Autodesk Fusion 360 part; units mm, degrees
note: some values were not read from the file. Set by a fixed rule: which sketch regions a step uses.
(part 4 of 4)
  line L683 (3.4369, -40.79) -> (3.9769, -40.4465)
  line L684 (3.9769, -40.4465) -> (3.9994, -40.4318)
  line L685 (3.9994, -40.4318) -> (4.2354, -40.3019)
  line L686 (4.2354, -40.3019) -> (4.2599, -40.2908)
  line L687 (4.2599, -40.2908) -> (4.2279, -40.2967)
  line L688 (4.2279, -40.2967) -> (3.9619, -40.3254)
  line L689 (3.9619, -40.3254) -> (3.4369, -40.3254)
  line L690 (3.4369, -40.3254) -> (3.4369, -39.957)
  line L691 (3.4369, -39.957) -> (4.9125, -39.9578)
  line L692 (4.9125, -39.9578) -> (4.9125, -40.3262)
  line L693 (4.9125, -40.3262) -> (4.2619, -40.7299)
  line L694 (4.2619, -40.7299) -> (4.2373, -40.7447)
  line L695 (4.2373, -40.7447) -> (3.9836, -40.8754)
  line L696 (3.777, -41.5549) -> (3.777, -42.2201)
  line L697 (3.777, -42.2201) -> (3.9912, -42.2201)
  line L698 (3.9912, -42.2201) -> (3.9912, -41.6824)
  line L699 (3.9912, -41.6824) -> (4.3186, -41.6824)
  line L700 (4.3186, -41.6824) -> (4.3186, -42.2201)
  line L701 (4.3186, -42.2201) -> (4.5619, -42.2201)
  line L702 (4.5619, -42.2201) -> (4.5619, -41.5549)
  line L703 (4.5619, -41.5549) -> (4.9141, -41.5549)
  line L704 (4.9141, -41.5549) -> (4.9141, -42.665)
  line L705 (4.9141, -42.665) -> (3.4369, -42.665)
  line L706 (3.4369, -42.665) -> (3.4369, -41.5549)
  line L707 (3.4369, -41.5549) -> (3.777, -41.5549)
  line L708 (4.9125, -44.0314) -> (3.4369, -44.0314)
  line L709 (3.4369, -44.0314) -> (3.4369, -42.965)
  line L710 (3.4369, -42.965) -> (3.7879, -42.965)
  line L711 (3.7879, -42.965) -> (3.7879, -43.5908)
  line L712 (3.7879, -43.5908) -> (4.0279, -43.5908)
  line L713 (4.0279, -43.5908) -> (4.0279, -43.1102)
  line L714 (4.0279, -43.1102) -> (4.3606, -43.1102)
  line L715 (4.3606, -43.1102) -> (4.3606, -43.5908)
  line L716 (4.3606, -43.5908) -> (4.9125, -43.5908)
  line L717 (4.9125, -43.5908) -> (4.9125, -44.0314)
  line L718 (4.2994, -45.1875) -> (4.2994, -44.949)
  line L719 (4.2994, -44.949) -> (3.8715, -45.0684)
  line L720 (3.8715, -45.0684) -> (4.2994, -45.1875)
  line L721 (4.9125, -44.7863) -> (4.6219, -44.8695)
  line L722 (4.6219, -44.8695) -> (4.6219, -45.2648)
  line L723 (4.6219, -45.2648) -> (4.9125, -45.3533)
  line L724 (4.9125, -45.3533) -> (4.9125, -45.7209)
  line L725 (4.9125, -45.7209) -> (3.4369, -45.2656)
  line L726 (3.4369, -45.2656) -> (3.4369, -44.7867)
  line L727 (3.4369, -44.7867) -> (4.9113, -44.3244)
  line L728 (4.9113, -44.3244) -> (4.9125, -44.7863)
  line L729 (3.9791, -46.4652) -> (3.4369, -46.4652)
  line L730 (3.4369, -46.4652) -> (3.4369, -46.0125)
  line L731 (3.4369, -46.0125) -> (4.9113, -46.0125)
  line L732 (4.9113, -46.0125) -> (4.9113, -46.4652)
  line L733 (4.9113, -46.4652) -> (4.3393, -46.4652)
  line L734 (4.3393, -46.4652) -> (4.3393, -46.8109)
  line L735 (4.3393, -46.8109) -> (4.9125, -46.8109)
  line L736 (4.9125, -46.8109) -> (4.9125, -47.2637)
  line L737 (4.9125, -47.2637) -> (3.4369, -47.2637)
  line L738 (3.4369, -47.2637) -> (3.4369, -46.8109)
  line L739 (3.4369, -46.8109) -> (3.9791, -46.8109)
  line L740 (3.9791, -46.8109) -> (3.9791, -46.4652)
  line L741 (4.0338, -48.2893) -> (4.0039, -48.1742)
  line L742 (4.0039, -48.1742) -> (3.9975, -48.1639)
  line L743 (3.9975, -48.1639) -> (3.9916, -48.1553)
  line L744 (3.9916, -48.1553) -> (3.952, -48.1244)
  line L745 (3.952, -48.1244) -> (3.9033, -48.1117)
  line L746 (3.9033, -48.1117) -> (3.893, -48.1121)
  line L747 (3.893, -48.1121) -> (3.8662, -48.1121)
  line L748 (3.8662, -48.1121) -> (3.7865, -48.1557)
  line L749 (3.7865, -48.1557) -> (3.7512, -48.2533)
  line L750 (3.7512, -48.2533) -> (3.7512, -48.4943)
  line L751 (3.7512, -48.4943) -> (4.0332, -48.4943)
  line L752 (4.0332, -48.4943) -> (4.0332, -48.3012)
  line L753 (4.0332, -48.3012) -> (4.0338, -48.2893)
  line L754 (3.4369, -48.1211) -> (3.4666, -47.9514)
  line L755 (3.4666, -47.9514) -> (3.5363, -47.8055)
  line L756 (3.5363, -47.8055) -> (3.5563, -47.7818)
  line L757 (3.5563, -47.7818) -> (3.5755, -47.7586)
  line L758 (3.5755, -47.7586) -> (3.6973, -47.6748)
  line L759 (3.6973, -47.6748) -> (3.8408, -47.6398)
  line L760 (3.8408, -47.6398) -> (3.8711, -47.6408)
  line L761 (3.8711, -47.6408) -> (3.8906, -47.6404)
  line L762 (3.8906, -47.6404) -> (4.0787, -47.6838)
  line L763 (4.0787, -47.6838) -> (4.0961, -47.6926)
  line L764 (4.0961, -47.6926) -> (4.1123, -47.7014)
  line L765 (4.1123, -47.7014) -> (4.1879, -47.7709)
  line L766 (4.1879, -47.7709) -> (4.2559, -47.876)
  line L767 (4.2559, -47.876) -> (4.2684, -47.9021)
  line L768 (4.2684, -47.9021) -> (4.9125, -47.6344)
  line L769 (4.9125, -47.6344) -> (4.9125, -48.1361)
  line L770 (4.9125, -48.1361) -> (4.35, -48.3518)
  line L771 (4.35, -48.3518) -> (4.35, -48.4943)
  line L772 (4.35, -48.4943) -> (4.9125, -48.4943)
  line L773 (4.9125, -48.4943) -> (4.9125, -48.9469)
  line L774 (4.9125, -48.9469) -> (3.4369, -48.9469)
  line L775 (3.4369, -48.9469) -> (3.4369, -48.1211)
  line L776 (3.9912, -49.4111) -> (4.3186, -49.4111)
  line L777 (4.3186, -49.4111) -> (4.3186, -49.949)
  line L778 (4.3186, -49.949) -> (4.5619, -49.949)
  line L779 (4.5619, -49.949) -> (4.5619, -49.2838)
  line L780 (4.5619, -49.2838) -> (4.9141, -49.2838)
  line L781 (4.9141, -49.2838) -> (4.9141, -50.393)
  line L782 (4.9141, -50.393) -> (3.4369, -50.393)
  line L783 (3.4369, -50.393) -> (3.4369, -49.2838)
  line L784 (3.4369, -49.2838) -> (3.777, -49.2838)
  line L785 (3.777, -49.2838) -> (3.777, -49.949)
  line L786 (3.777, -49.949) -> (3.9912, -49.949)
  line L787 (3.9912, -49.949) -> (3.9912, -49.4111)
  line L788 (4.9125, -51.5742) -> (4.9125, -52.0025)
  line L789 (4.9125, -52.0025) -> (3.4369, -52.0025)
  line L790 (3.4369, -52.0025) -> (3.4369, -51.5758)
  line L791 (3.4369, -51.5758) -> (4.0467, -51.5758)
  line L792 (4.0467, -51.5758) -> (3.4369, -51.1678)
  line L793 (3.4369, -51.1678) -> (3.4369, -50.7607)
  line L794 (3.4369, -50.7607) -> (3.9766, -51.1332)
  line L795 (3.9766, -51.1332) -> (4.9125, -50.6713)
  line L796 (4.9125, -50.6713) -> (4.9125, -51.1666)
  line L797 (4.9125, -51.1666) -> (4.3553, -51.4213)
  line L798 (4.3553, -51.4213) -> (4.5725, -51.5742)
  line L799 (4.5725, -51.5742) -> (4.9125, -51.5742)
  line L800 (4.2994, -53.1574) -> (4.2994, -52.9185)
  line L801 (4.2994, -52.9185) -> (3.8715, -53.0379)
  line L802 (3.8715, -53.0379) -> (4.2994, -53.1574)
  line L803 (4.6219, -52.8391) -> (4.6219, -53.2344)
  line L804 (4.6219, -53.2344) -> (4.9125, -53.3228)
  line L805 (4.9125, -53.3228) -> (4.9125, -53.69)
  line L806 (4.9125, -53.69) -> (3.4369, -53.2352)
  line L807 (3.4369, -53.2352) -> (3.4369, -52.7566)
  line L808 (3.4369, -52.7566) -> (4.9113, -52.2937)
  line L809 (4.9113, -52.2937) -> (4.9125, -52.7559)
  line L810 (4.9125, -52.7559) -> (4.6219, -52.8391)
  line L811 (3.8584, -54.4025) -> (4.9125, -54.675)
  line L812 (4.9125, -54.675) -> (4.9125, -54.965)
  line L813 (4.9125, -54.965) -> (3.8584, -55.2488)
  line L814 (3.8584, -55.2488) -> (4.9125, -55.2488)
  line L815 (4.9125, -55.2488) -> (4.9125, -55.5863)
  line L816 (4.9125, -55.5863) -> (3.4369, -55.5863)
  line L817 (3.4369, -55.5863) -> (3.4369, -54.9949)
  line L818 (3.4369, -54.9949) -> (4.2203, -54.7809)
  line L819 (4.2203, -54.7809) -> (3.4369, -54.5768)
  line L820 (3.4369, -54.5768) -> (3.4369, -53.9832)
  line L821 (3.4369, -53.9832) -> (4.9113, -53.9832)
  line L822 (4.9113, -53.9832) -> (4.9113, -54.4025)
  line L823 (4.9113, -54.4025) -> (3.8584, -54.4025)
  dimension "d75" = 5
sketch "Sketch1 (2)" plane through (0, 0, 0) normal (0, 1, 0) x (1, 0, 0) in component "Teller"
  line L0 (10, 0) -> (10, -6.3694)
  line L1 (1.5, -1.5) -> (1.5, 0)
  line L2 (0, 0) -> (10, 0)
  line L3 (10, -6.3694) -> (9, -6.3694)
  line L4 (0, -1.5) -> (9, -1.5)
  line L5 (9, -1.5) -> (9, -6.3694)
  line L6 (0, 0) -> (0, -1.5)
  dimension "d49" = 1.5
  dimension "d50" = 10
  dimension "d51" = 6.3694
  dimension "d52" = 1
  dimension "d11" = 1.5
  constraint coincident L2.start L6.start
  constraint horizontal L2
  constraint perpendicular L0 L2
  constraint perpendicular L0 L3
  constraint perpendicular L2 L6
  constraint perpendicular L0 L4
  constraint perpendicular L3 L5
  constraint coincident L1.start L4
  constraint coincident L1.end L2
  constraint perpendicular L1 L2
  measures "d49" distance of L1 L6
  measures "d50" distance of L0.start L2.start
  measures "d51" distance of L0.start L0.end
  measures "d52" distance of L3.end L0.end
  measures "d11" distance of L4.start L2.start
revolve "Revolve1" add sketch "Sketch1 (2)" angle 360 about axis through (0, 0, 1.75) along (0, 0, 1) separate body contours L0 L1 L2 L3 L4 L5 makes body 6 in component "Teller"
fillet "Fillet1'''" radius 3.5 2 edges at (-9.3233, -3.6162, 0) (-8.3909, -3.2545, 1.5) on bodies 6 in component "Teller"
fillet "Fillet2" radius 0.5 2 edges at (-9.3233, -3.6162, 6.3694) (-8.3909, -3.2545, 6.3694) on bodies 6 in component "Teller"
chamfer "Chamfer1" distance 1.25 angle 45 1 edges at (-1.3985, -0.5424, 1.5) on bodies 6 in component "Teller"
component "Boden" placed x (1, 0, 0) y (0, 1, 0) z (0, 0, 1) at (-162.7017, 0, -2.5423)
component "Halter" placed x (0, 0, 1) y (0, -1, 0) z (1, 0, 0) at (42.7603, -3.5, -195.5112)
component "Seite" placed x (0, -1, 0) y (-1, 0, 0) z (0, 0, -1) at (-0.7017, 8, -112.5423)
component "Hebel" placed x (1, 0, 0) y (0, 1, 0) z (0, 0, 1) at (-97.7017, -38.5, -2.5423)
component "Quer" placed x (0, -1, 0) y (0, 0, -1) z (1, 0, 0) at (24.8863, 163.6643, -36.5423)
component "Seite" placed x (0, -1, 0) y (-1, 0, 0) z (0, 0, -1) at (-55.7017, 8, -112.5423)
component "Laser" placed x (1, 0, 0) y (0, 1, 0) z (0, 0, 1) at (0, 0, 0)
component "Teller" placed x (1, 0, 0) y (0, 0, 1) z (0, -1, 0) at (-30.7017, -38.5, -92.8071)
equation "d50 = durchmesser / 2"
equation "d51 = hoehe"
equation "durchmesser = 20 mm"
equation "hoehe = durchmesser / 3.14"
